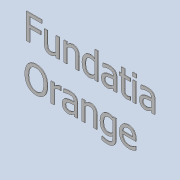
# Autodesk Inventor part: Fundatia orange
Saved by Autodesk Inventor 2020 (Build 240168000, 168)
## iProperties
Created: 2021-01-22
Part Number: Fundatia orange
Material: Generic
Document SubType Name: Modeling
Designer: Iulian Bors
Density: 1 g/cm^3
Appearance: Default
Author: Iulian Bors
Autodesk Inventor part; units mm, degrees
ref_plane "YZ Plane" through (0, 0, 0) normal (1, 0, 0) x (0, 1, 0)
ref_plane "XZ Plane" through (0, 0, 0) normal (0, 1, 0) x (-1, 0, 0)
ref_plane "XY Plane" through (0, 0, 0) normal (0, 0, 1) x (1, 0, 0)
sketch "Sketch1" plane through (0, 0, 0) normal (0, 0, 1) x (1, 0, 0)
  line L0 (-100, 150) -> (100, 150)
  line L1 (100, 150) -> (100, -150)
  line L2 (100, -150) -> (-100, -150)
  line L3 (-100, -150) -> (-100, 150)
  line L4 (-64.214, 58.4793) -> (-50.2905, 58.4793) construction
  line L5 (-50.2905, 58.4793) -> (-50.2905, 44.5299) construction
  line L6 (-50.2905, 44.5299) -> (-64.214, 44.5299) construction
  line L7 (-64.214, 44.5299) -> (-64.214, 58.4793) construction
  line L8 (-25, -80) -> (25, -80)
  line L9 (25, -80) -> (25, -130)
  line L10 (25, -130) -> (-25, -130)
  line L11 (-25, -130) -> (-25, -80)
  line L12 (-46.7302, 54.4072) -> (-58.359, 54.4072)
  line L13 (-58.359, 54.4072) -> (-58.359, 47.357)
  line L14 (-58.359, 47.357) -> (-47.2164, 47.357)
  line L15 (-47.2164, 47.357) -> (-47.2164, 44.3991)
  line L16 (-47.2164, 44.3991) -> (-58.359, 44.3991)
  line L17 (-58.359, 44.3991) -> (-58.359, 32.3651)
  line L18 (-58.359, 32.3651) -> (-61.6815, 32.3651)
  line L19 (-61.6815, 32.3651) -> (-61.6815, 57.3651)
  line L20 (-61.6815, 57.3651) -> (-46.7302, 57.3651)
  line L21 (-46.7302, 57.3651) -> (-46.7302, 54.4072)
  line L22 (-29.4084, 32.3651) -> (-32.5689, 32.3651)
  line L23 (-32.5689, 32.3651) -> (-32.5689, 34.4315)
  spline S0 degree 2 poles (-32.5689, 34.4315) (-34.0276, 33.1552) (-36.641, 31.8383) (-38.2618, 31.8383) knots 0 0 0 1 2 2 2
  spline S1 degree 2 poles (-38.2618, 31.8383) (-39.4773, 31.8383) (-41.6451, 32.6487) (-42.4352, 33.5199) knots 0 0 0 1 2 2 2
  spline S2 degree 2 poles (-42.4352, 33.5199) (-43.2456, 34.391) (-44.137, 37.045) (-44.137, 38.9494) knots 0 0 0 1 2 2 2
  line L24 (-44.137, 38.9494) -> (-44.137, 51.1252)
  line L25 (-44.137, 51.1252) -> (-40.9765, 51.1252)
  line L26 (-40.9765, 51.1252) -> (-40.9765, 40.4283)
  spline S3 degree 2 poles (-40.9765, 40.4283) (-40.9765, 38.9291) (-40.7537, 36.9639) (-40.3687, 36.2346) knots 0 0 0 1 2 2 2
  spline S4 degree 2 poles (-40.3687, 36.2346) (-39.9838, 35.5053) (-38.667, 34.8367) (-37.4311, 34.8367) knots 0 0 0 1 2 2 2
  spline S5 degree 2 poles (-37.4311, 34.8367) (-36.2764, 34.8367) (-33.6629, 36.1536) (-32.5689, 37.1058) knots 0 0 0 1 2 2 2
  line L27 (-32.5689, 37.1058) -> (-32.5689, 51.1252)
  line L28 (-32.5689, 51.1252) -> (-29.4084, 51.1252)
  line L29 (-29.4084, 51.1252) -> (-29.4084, 32.3651)
  line L30 (-10.1013, 32.3651) -> (-13.2618, 32.3651)
  line L31 (-13.2618, 32.3651) -> (-13.2618, 43.062)
  spline S6 degree 2 poles (-13.2618, 43.062) (-13.2618, 44.3586) (-13.5049, 46.5871) (-13.8696, 47.2557) knots 0 0 0 1 2 2 2
  spline S7 degree 2 poles (-13.8696, 47.2557) (-14.2545, 47.9648) (-15.6321, 48.6536) (-16.8072, 48.6536) knots 0 0 0 1 2 2 2
  spline S8 degree 2 poles (-16.8072, 48.6536) (-17.9822, 48.6536) (-20.4741, 47.3975) (-21.6694, 46.3845) knots 0 0 0 1 2 2 2
  line L32 (-21.6694, 46.3845) -> (-21.6694, 32.3651)
  line L33 (-21.6694, 32.3651) -> (-24.8298, 32.3651)
  line L34 (-24.8298, 32.3651) -> (-24.8298, 51.1252)
  line L35 (-24.8298, 51.1252) -> (-21.6694, 51.1252)
  line L36 (-21.6694, 51.1252) -> (-21.6694, 49.0385)
  spline S9 degree 2 poles (-21.6694, 49.0385) (-20.2512, 50.3148) (-17.5162, 51.652) (-15.9765, 51.652) knots 0 0 0 1 2 2 2
  spline S10 degree 2 poles (-15.9765, 51.652) (-13.2213, 51.652) (-10.1013, 48.0053) (-10.1013, 44.5409) knots 0 0 0 1 2 2 2
  line L37 (-10.1013, 44.5409) -> (-10.1013, 32.3651)
  line L38 (8.7601, 32.3651) -> (5.5997, 32.3651)
  line L39 (5.5997, 32.3651) -> (5.5997, 34.2695)
  spline S11 degree 2 poles (5.5997, 34.2695) (4.8703, 33.6617) (3.7966, 32.8513) (3.0672, 32.5069) knots 0 0 0 1 2 2 2
  spline S12 degree 2 poles (3.0672, 32.5069) (2.3987, 32.1827) (0.9603, 31.8383) (0.0081, 31.8383) knots 0 0 0 1 2 2 2
  spline S13 degree 2 poles (0.0081, 31.8383) (-1.5316, 31.8383) (-4.1248, 33.1147) (-5.0365, 34.3505) knots 0 0 0 1 2 2 2
  spline S14 degree 2 poles (-5.0365, 34.3505) (-5.9482, 35.5863) (-6.9611, 39.233) (-6.9611, 41.6033) knots 0 0 0 1 2 2 2
  spline S15 degree 2 poles (-6.9611, 41.6033) (-6.9611, 44.075) (-5.6848, 47.6811) (-4.5705, 49.0385) knots 0 0 0 1 2 2 2
  spline S16 degree 2 poles (-4.5705, 49.0385) (-3.5373, 50.2541) (-0.6402, 51.652) (0.9603, 51.652) knots 0 0 0 1 2 2 2
  spline S17 degree 2 poles (0.9603, 51.652) (2.3582, 51.652) (4.4449, 51.0239) (5.5997, 50.3756) knots 0 0 0 1 2 2 2
  line L40 (5.5997, 50.3756) -> (5.5997, 58.4793)
  line L41 (5.5997, 58.4793) -> (8.7601, 58.4793)
  line L42 (8.7601, 58.4793) -> (8.7601, 32.3651)
  line L43 (5.5997, 36.9234) -> (5.5997, 47.7622)
  spline S18 degree 2 poles (5.5997, 47.7622) (4.4246, 48.3294) (2.5608, 48.7549) (1.487, 48.7549) knots 0 0 0 1 2 2 2
  spline S19 degree 2 poles (1.487, 48.7549) (-0.9441, 48.7549) (-3.6994, 45.1082) (-3.6994, 41.6641) knots 0 0 0 1 2 2 2
  spline S20 degree 2 poles (-3.6994, 41.6641) (-3.6994, 38.3416) (-1.5924, 34.8367) (0.7374, 34.8367) knots 0 0 0 1 2 2 2
  spline S21 degree 2 poles (0.7374, 34.8367) (1.9732, 34.8367) (4.4854, 35.9712) (5.5997, 36.9234) knots 0 0 0 1 2 2 2
  spline S22 degree 2 poles (23.7925, 34.3505) (23.4076, 34.0669) (22.111, 33.0539) (21.5032, 32.75) knots 0 0 0 1 2 2 2
  spline S23 degree 2 poles (21.5032, 32.75) (20.6726, 32.3043) (19.1126, 31.8383) (17.6945, 31.8383) knots 0 0 0 1 2 2 2
  spline S24 degree 2 poles (17.6945, 31.8383) (16.5397, 31.8383) (14.453, 32.7095) (13.6629, 33.4996) knots 0 0 0 1 2 2 2
  spline S25 degree 2 poles (13.6629, 33.4996) (12.9133, 34.2695) (12.0016, 36.5385) (12.0016, 37.7946) knots 0 0 0 1 2 2 2
  spline S26 degree 2 poles (12.0016, 37.7946) (12.0016, 39.7395) (13.6426, 42.4947) (15.4254, 43.2849) knots 0 0 0 1 2 2 2
  spline S27 degree 2 poles (15.4254, 43.2849) (17.0057, 44.0142) (21.3006, 44.5612) (23.7925, 44.703) knots 0 0 0 1 2 2 2
  line L44 (23.7925, 44.703) -> (23.7925, 45.3108)
  spline S28 degree 2 poles (23.7925, 45.3108) (23.7925, 46.4048) (23.124, 47.7622) (22.5162, 48.1471) knots 0 0 0 1 2 2 2
  spline S29 degree 2 poles (22.5162, 48.1471) (21.9084, 48.532) (20.1661, 48.7751) (19.2342, 48.7751) knots 0 0 0 1 2 2 2
  spline S30 degree 2 poles (19.2342, 48.7751) (18.1402, 48.7751) (15.1823, 48.1268) (13.7034, 47.4988) knots 0 0 0 1 2 2 2
  line L45 (13.7034, 47.4988) -> (13.521, 47.4988)
  line L46 (13.521, 47.4988) -> (13.521, 50.72)
  spline S31 degree 2 poles (13.521, 50.72) (14.3922, 50.9631) (17.6539, 51.5709) (19.2544, 51.5709) knots 0 0 0 1 2 2 2
  spline S32 degree 2 poles (19.2544, 51.5709) (21.1993, 51.5709) (23.8533, 50.9631) (24.9068, 50.173) knots 0 0 0 1 2 2 2
  spline S33 degree 2 poles (24.9068, 50.173) (25.94, 49.4032) (26.953, 46.9518) (26.953, 45.1892) knots 0 0 0 1 2 2 2
  line L47 (26.953, 45.1892) -> (26.953, 32.3651)
  line L48 (26.953, 32.3651) -> (23.7925, 32.3651)
  line L49 (23.7925, 32.3651) -> (23.7925, 34.3505)
  line L50 (23.7925, 36.9842) -> (23.7925, 42.1908)
  spline S34 degree 2 poles (23.7925, 42.1908) (22.658, 42.0896) (19.2342, 41.7451) (18.1604, 41.421) knots 0 0 0 1 2 2 2
  spline S35 degree 2 poles (18.1604, 41.421) (16.9044, 41.0361) (15.2634, 39.4356) (15.2634, 38.0174) knots 0 0 0 1 2 2 2
  spline S36 degree 2 poles (15.2634, 38.0174) (15.2634, 36.3967) (17.0867, 34.7557) (18.829, 34.7557) knots 0 0 0 1 2 2 2
  spline S37 degree 2 poles (18.829, 34.7557) (20.3079, 34.7557) (22.739, 36.032) (23.7925, 36.9842) knots 0 0 0 1 2 2 2
  spline S38 degree 2 poles (37.0624, 32.0004) (34.4894, 32.0004) (31.5924, 34.938) (31.5924, 38.1187) knots 0 0 0 1 2 2 2
  line L51 (31.5924, 38.1187) -> (31.5924, 48.5118)
  line L52 (31.5924, 48.5118) -> (29.4651, 48.5118)
  line L53 (29.4651, 48.5118) -> (29.4651, 51.1252)
  line L54 (29.4651, 51.1252) -> (31.5924, 51.1252)
  line L55 (31.5924, 51.1252) -> (31.5924, 56.5142)
  line L56 (31.5924, 56.5142) -> (34.7528, 56.5142)
  line L57 (34.7528, 56.5142) -> (34.7528, 51.1252)
  line L58 (34.7528, 51.1252) -> (40.5672, 51.1252)
  line L59 (40.5672, 51.1252) -> (40.5672, 48.5118)
  line L60 (40.5672, 48.5118) -> (34.7528, 48.5118)
  line L61 (34.7528, 48.5118) -> (34.7528, 39.5774)
  spline S39 degree 2 poles (34.7528, 39.5774) (34.7528, 38.1592) (34.8541, 36.5993) (35.1985, 35.9307) knots 0 0 0 1 2 2 2
  spline S40 degree 2 poles (35.1985, 35.9307) (35.4822, 35.3432) (36.7585, 34.7557) (37.8525, 34.7557) knots 0 0 0 1 2 2 2
  spline S41 degree 2 poles (37.8525, 34.7557) (38.6223, 34.7557) (40.0608, 35.2216) (40.3849, 35.3635) knots 0 0 0 1 2 2 2
  line L62 (40.3849, 35.3635) -> (40.5672, 35.3635)
  line L63 (40.5672, 35.3635) -> (40.5672, 32.5272)
  spline S42 degree 2 poles (40.5672, 32.5272) (39.6758, 32.284) (37.8525, 32.0004) (37.0624, 32.0004) knots 0 0 0 1 2 2 2
  line L64 (46.1183, 32.3651) -> (42.9578, 32.3651)
  line L65 (42.9578, 32.3651) -> (42.9578, 51.1252)
  line L66 (42.9578, 51.1252) -> (46.1183, 51.1252)
  line L67 (46.1183, 51.1252) -> (46.1183, 32.3651)
  line L68 (46.3411, 54.2451) -> (42.7552, 54.2451)
  line L69 (42.7552, 54.2451) -> (42.7552, 57.5272)
  line L70 (42.7552, 57.5272) -> (46.3411, 57.5272)
  line L71 (46.3411, 57.5272) -> (46.3411, 54.2451)
  spline S43 degree 2 poles (61.2115, 34.3505) (60.8266, 34.0669) (59.53, 33.0539) (58.9222, 32.75) knots 0 0 0 1 2 2 2
  spline S44 degree 2 poles (58.9222, 32.75) (58.0916, 32.3043) (56.5316, 31.8383) (55.1134, 31.8383) knots 0 0 0 1 2 2 2
  spline S45 degree 2 poles (55.1134, 31.8383) (53.9586, 31.8383) (51.8719, 32.7095) (51.0818, 33.4996) knots 0 0 0 1 2 2 2
  spline S46 degree 2 poles (51.0818, 33.4996) (50.3322, 34.2695) (49.4206, 36.5385) (49.4206, 37.7946) knots 0 0 0 1 2 2 2
  spline S47 degree 2 poles (49.4206, 37.7946) (49.4206, 39.7395) (51.0616, 42.4947) (52.8444, 43.2849) knots 0 0 0 1 2 2 2
  spline S48 degree 2 poles (52.8444, 43.2849) (54.4246, 44.0142) (58.7196, 44.5612) (61.2115, 44.703) knots 0 0 0 1 2 2 2
  line L72 (61.2115, 44.703) -> (61.2115, 45.3108)
  spline S49 degree 2 poles (61.2115, 45.3108) (61.2115, 46.4048) (60.5429, 47.7622) (59.9351, 48.1471) knots 0 0 0 1 2 2 2
  spline S50 degree 2 poles (59.9351, 48.1471) (59.3274, 48.532) (57.5851, 48.7751) (56.6531, 48.7751) knots 0 0 0 1 2 2 2
  spline S51 degree 2 poles (56.6531, 48.7751) (55.5591, 48.7751) (52.6013, 48.1268) (51.1223, 47.4988) knots 0 0 0 1 2 2 2
  line L73 (51.1223, 47.4988) -> (50.94, 47.4988)
  line L74 (50.94, 47.4988) -> (50.94, 50.72)
  spline S52 degree 2 poles (50.94, 50.72) (51.8112, 50.9631) (55.0729, 51.5709) (56.6734, 51.5709) knots 0 0 0 1 2 2 2
  spline S53 degree 2 poles (56.6734, 51.5709) (58.6183, 51.5709) (61.2723, 50.9631) (62.3257, 50.173) knots 0 0 0 1 2 2 2
  spline S54 degree 2 poles (62.3257, 50.173) (63.359, 49.4032) (64.3719, 46.9518) (64.3719, 45.1892) knots 0 0 0 1 2 2 2
  line L75 (64.3719, 45.1892) -> (64.3719, 32.3651)
  line L76 (64.3719, 32.3651) -> (61.2115, 32.3651)
  line L77 (61.2115, 32.3651) -> (61.2115, 34.3505)
  line L78 (61.2115, 36.9842) -> (61.2115, 42.1908)
  spline S55 degree 2 poles (61.2115, 42.1908) (60.077, 42.0896) (56.6531, 41.7451) (55.5794, 41.421) knots 0 0 0 1 2 2 2
  spline S56 degree 2 poles (55.5794, 41.421) (54.3233, 41.0361) (52.6823, 39.4356) (52.6823, 38.0174) knots 0 0 0 1 2 2 2
  spline S57 degree 2 poles (52.6823, 38.0174) (52.6823, 36.3967) (54.5057, 34.7557) (56.248, 34.7557) knots 0 0 0 1 2 2 2
  spline S58 degree 2 poles (56.248, 34.7557) (57.7269, 34.7557) (60.158, 36.032) (61.2115, 36.9842) knots 0 0 0 1 2 2 2
  spline S59 degree 2 poles (-43.9952, 13.3467) (-42.577, 11.6854) (-40.9968, 6.8232) (-40.9968, 3.7032) knots 0 0 0 1 2 2 2
  spline S60 degree 2 poles (-40.9968, 3.7032) (-40.9968, 0.6643) (-42.5365, -4.2587) (-43.9952, -5.9199) knots 0 0 0 1 2 2 2
  spline S61 degree 2 poles (-43.9952, -5.9199) (-45.5349, -7.6622) (-49.607, -9.3235) (-52.0584, -9.3235) knots 0 0 0 1 2 2 2
  spline S62 degree 2 poles (-52.0584, -9.3235) (-54.5908, -9.3235) (-58.6426, -7.6015) (-60.1216, -5.9199) knots 0 0 0 1 2 2 2
  spline S63 degree 2 poles (-60.1216, -5.9199) (-61.56, -4.2587) (-63.0997, 0.6238) (-63.0997, 3.7032) knots 0 0 0 1 2 2 2
  spline S64 degree 2 poles (-63.0997, 3.7032) (-63.0997, 6.8434) (-61.5397, 11.6246) (-60.1013, 13.3467) knots 0 0 0 1 2 2 2
  spline S65 degree 2 poles (-60.1013, 13.3467) (-58.6426, 15.0079) (-54.5705, 16.73) (-52.0584, 16.73) knots 0 0 0 1 2 2 2
  spline S66 degree 2 poles (-52.0584, 16.73) (-49.5057, 16.73) (-45.4133, 14.9472) (-43.9952, 13.3467) knots 0 0 0 1 2 2 2
  spline S67 degree 2 poles (-44.4611, 3.7032) (-44.4611, 6.1749) (-45.5349, 10.0039) (-46.5073, 11.26) knots 0 0 0 1 2 2 2
  spline S68 degree 2 poles (-46.5073, 11.26) (-47.5, 12.5566) (-50.2958, 13.8532) (-52.0381, 13.8532) knots 0 0 0 1 2 2 2
  spline S69 degree 2 poles (-52.0381, 13.8532) (-53.8412, 13.8532) (-56.5559, 12.5971) (-57.5892, 11.26) knots 0 0 0 1 2 2 2
  spline S70 degree 2 poles (-57.5892, 11.26) (-58.5819, 9.9836) (-59.6354, 6.1344) (-59.6354, 3.7032) knots 0 0 0 1 2 2 2
  spline S71 degree 2 poles (-59.6354, 3.7032) (-59.6354, -1.2198) (-55.5025, -6.4467) (-52.0381, -6.4467) knots 0 0 0 1 2 2 2
  spline S72 degree 2 poles (-52.0381, -6.4467) (-48.5738, -6.4467) (-44.4611, -1.2198) (-44.4611, 3.7032) knots 0 0 0 1 2 2 2
  line L79 (-27.6459, 6.5801) -> (-27.808, 6.5801)
  spline S73 degree 2 poles (-27.808, 6.5801) (-28.1726, 6.6814) (-28.9627, 6.7219) (-29.5097, 6.7219) knots 0 0 0 1 2 2 2
  spline S74 degree 2 poles (-29.5097, 6.7219) (-30.7861, 6.7219) (-33.2982, 5.6076) (-34.4328, 4.5136) knots 0 0 0 1 2 2 2
  line L80 (-34.4328, 4.5136) -> (-34.4328, -8.7968)
  line L81 (-34.4328, -8.7968) -> (-37.5932, -8.7968)
  line L82 (-37.5932, -8.7968) -> (-37.5932, 9.9634)
  line L83 (-37.5932, 9.9634) -> (-34.4328, 9.9634)
  line L84 (-34.4328, 9.9634) -> (-34.4328, 7.1676)
  spline S75 degree 2 poles (-34.4328, 7.1676) (-32.7107, 8.7073) (-30.1378, 9.9634) (-28.9222, 9.9634) knots 0 0 0 1 2 2 2
  spline S76 degree 2 poles (-28.9222, 9.9634) (-28.436, 9.9634) (-27.9498, 9.9228) (-27.6459, 9.8621) knots 0 0 0 1 2 2 2
  line L85 (-27.6459, 9.8621) -> (-27.6459, 6.5801)
  spline S77 degree 2 poles (-14.7407, -6.8113) (-15.1256, -7.095) (-16.4222, -8.1079) (-17.03, -8.4118) knots 0 0 0 1 2 2 2
  spline S78 degree 2 poles (-17.03, -8.4118) (-17.8606, -8.8575) (-19.4206, -9.3235) (-20.8388, -9.3235) knots 0 0 0 1 2 2 2
  spline S79 degree 2 poles (-20.8388, -9.3235) (-21.9935, -9.3235) (-24.0802, -8.4524) (-24.8704, -7.6622) knots 0 0 0 1 2 2 2
  spline S80 degree 2 poles (-24.8704, -7.6622) (-25.62, -6.8924) (-26.5316, -4.6233) (-26.5316, -3.3673) knots 0 0 0 1 2 2 2
  spline S81 degree 2 poles (-26.5316, -3.3673) (-26.5316, -1.4224) (-24.8906, 1.3329) (-23.1078, 2.123) knots 0 0 0 1 2 2 2
  spline S82 degree 2 poles (-23.1078, 2.123) (-21.5276, 2.8523) (-17.2326, 3.3993) (-14.7407, 3.5412) knots 0 0 0 1 2 2 2
  line L86 (-14.7407, 3.5412) -> (-14.7407, 4.1489)
  spline S83 degree 2 poles (-14.7407, 4.1489) (-14.7407, 5.2429) (-15.4093, 6.6003) (-16.017, 6.9852) knots 0 0 0 1 2 2 2
  spline S84 degree 2 poles (-16.017, 6.9852) (-16.6248, 7.3702) (-18.3671, 7.6133) (-19.299, 7.6133) knots 0 0 0 1 2 2 2
  spline S85 degree 2 poles (-19.299, 7.6133) (-20.3931, 7.6133) (-23.3509, 6.965) (-24.8298, 6.3369) knots 0 0 0 1 2 2 2
  line L87 (-24.8298, 6.3369) -> (-25.0122, 6.3369)
  line L88 (-25.0122, 6.3369) -> (-25.0122, 9.5582)
  spline S86 degree 2 poles (-25.0122, 9.5582) (-24.141, 9.8013) (-20.8793, 10.4091) (-19.2788, 10.4091) knots 0 0 0 1 2 2 2
  spline S87 degree 2 poles (-19.2788, 10.4091) (-17.3339, 10.4091) (-14.6799, 9.8013) (-13.6264, 9.0112) knots 0 0 0 1 2 2 2
  spline S88 degree 2 poles (-13.6264, 9.0112) (-12.5932, 8.2413) (-11.5802, 5.7899) (-11.5802, 4.0274) knots 0 0 0 1 2 2 2
  line L89 (-11.5802, 4.0274) -> (-11.5802, -8.7968)
  line L90 (-11.5802, -8.7968) -> (-14.7407, -8.7968)
  line L91 (-14.7407, -8.7968) -> (-14.7407, -6.8113)
  line L92 (-14.7407, -4.1776) -> (-14.7407, 1.029)
  spline S89 degree 2 poles (-14.7407, 1.029) (-15.8752, 0.9277) (-19.299, 0.5833) (-20.3728, 0.2592) knots 0 0 0 1 2 2 2
  spline S90 degree 2 poles (-20.3728, 0.2592) (-21.6289, -0.1258) (-23.2699, -1.7263) (-23.2699, -3.1444) knots 0 0 0 1 2 2 2
  spline S91 degree 2 poles (-23.2699, -3.1444) (-23.2699, -4.7652) (-21.4465, -6.4062) (-19.7042, -6.4062) knots 0 0 0 1 2 2 2
  spline S92 degree 2 poles (-19.7042, -6.4062) (-18.2253, -6.4062) (-15.7942, -5.1298) (-14.7407, -4.1776) knots 0 0 0 1 2 2 2
  line L93 (7.5851, -8.7968) -> (4.4246, -8.7968)
  line L94 (4.4246, -8.7968) -> (4.4246, 1.9002)
  spline S93 degree 2 poles (4.4246, 1.9002) (4.4246, 3.1968) (4.1815, 5.4253) (3.8168, 6.0938) knots 0 0 0 1 2 2 2
  spline S94 degree 2 poles (3.8168, 6.0938) (3.4319, 6.8029) (2.0543, 7.4917) (0.8792, 7.4917) knots 0 0 0 1 2 2 2
  spline S95 degree 2 poles (0.8792, 7.4917) (-0.2958, 7.4917) (-2.7877, 6.2357) (-3.983, 5.2227) knots 0 0 0 1 2 2 2
  line L95 (-3.983, 5.2227) -> (-3.983, -8.7968)
  line L96 (-3.983, -8.7968) -> (-7.1435, -8.7968)
  line L97 (-7.1435, -8.7968) -> (-7.1435, 9.9634)
  line L98 (-7.1435, 9.9634) -> (-3.983, 9.9634)
  line L99 (-3.983, 9.9634) -> (-3.983, 7.8767)
  spline S96 degree 2 poles (-3.983, 7.8767) (-2.5649, 9.153) (0.1702, 10.4901) (1.7099, 10.4901) knots 0 0 0 1 2 2 2
  spline S97 degree 2 poles (1.7099, 10.4901) (4.4651, 10.4901) (7.5851, 6.8434) (7.5851, 3.3791) knots 0 0 0 1 2 2 2
  line L100 (7.5851, 3.3791) -> (7.5851, -8.7968)
  spline S98 degree 2 poles (12.6904, -11.7951) (13.0146, -11.937) (14.2504, -12.3827) (15.0405, -12.565) knots 0 0 0 1 2 2 2
  spline S99 degree 2 poles (15.0405, -12.565) (15.9116, -12.7878) (17.3906, -13.0512) (18.2617, -13.0512) knots 0 0 0 1 2 2 2
  spline S100 degree 2 poles (18.2617, -13.0512) (19.7204, -13.0512) (21.7463, -12.2814) (22.3136, -11.5925) knots 0 0 0 1 2 2 2
  spline S101 degree 2 poles (22.3136, -11.5925) (22.8606, -10.9037) (23.286, -9.1007) (23.286, -7.9459) knots 0 0 0 1 2 2 2
  line L101 (23.286, -7.9459) -> (23.286, -6.3049)
  spline S102 degree 2 poles (23.286, -6.3049) (22.0097, -7.4191) (19.5583, -8.4726) (17.7147, -8.4726) knots 0 0 0 1 2 2 2
  spline S103 degree 2 poles (17.7147, -8.4726) (14.5138, -8.4726) (10.7253, -3.7117) (10.7253, 0.7656) knots 0 0 0 1 2 2 2
  spline S104 degree 2 poles (10.7253, 0.7656) (10.7253, 3.0955) (12.0421, 6.7016) (13.1361, 7.978) knots 0 0 0 1 2 2 2
  spline S105 degree 2 poles (13.1361, 7.978) (14.1896, 9.1733) (17.0867, 10.4901) (18.6264, 10.4901) knots 0 0 0 1 2 2 2
  spline S106 degree 2 poles (18.6264, 10.4901) (20.0851, 10.4901) (22.2123, 9.8013) (23.286, 9.1733) knots 0 0 0 1 2 2 2
  line L102 (23.286, 9.1733) -> (23.4684, 9.9634)
  line L103 (23.4684, 9.9634) -> (26.4465, 9.9634)
  line L104 (26.4465, 9.9634) -> (26.4465, -6.6493)
  spline S107 degree 2 poles (26.4465, -6.6493) (26.4465, -11.4305) (22.2933, -15.8875) (18.0186, -15.8875) knots 0 0 0 1 2 2 2
  spline S108 degree 2 poles (18.0186, -15.8875) (16.641, -15.8875) (13.7642, -15.4418) (12.5283, -15.0772) knots 0 0 0 1 2 2 2
  line L105 (12.5283, -15.0772) -> (12.5283, -11.7951)
  line L106 (12.5283, -11.7951) -> (12.6904, -11.7951)
  line L107 (23.286, -3.7117) -> (23.286, 6.6003)
  spline S109 degree 2 poles (23.286, 6.6003) (22.111, 7.1676) (20.1256, 7.6538) (19.1329, 7.6538) knots 0 0 0 1 2 2 2
  spline S110 degree 2 poles (19.1329, 7.6538) (16.7423, 7.6538) (13.987, 4.1287) (13.987, 0.8264) knots 0 0 0 1 2 2 2
  spline S111 degree 2 poles (13.987, 0.8264) (13.987, -2.2935) (16.0737, -5.5553) (18.4238, -5.5553) knots 0 0 0 1 2 2 2
  spline S112 degree 2 poles (18.4238, -5.5553) (19.6596, -5.5553) (22.2528, -4.5828) (23.286, -3.7117) knots 0 0 0 1 2 2 2
  spline S113 degree 2 poles (39.1693, -9.2222) (34.6718, -9.2222) (29.7285, -4.1776) (29.7285, 0.482) knots 0 0 0 1 2 2 2
  spline S114 degree 2 poles (29.7285, 0.482) (29.7285, 5.0606) (34.53, 10.4901) (38.3995, 10.4901) knots 0 0 0 1 2 2 2
  spline S115 degree 2 poles (38.3995, 10.4901) (40.1418, 10.4901) (42.8363, 9.4771) (43.829, 8.4034) knots 0 0 0 1 2 2 2
  spline S116 degree 2 poles (43.829, 8.4034) (44.842, 7.3297) (45.9157, 4.23) (45.9157, 1.9812) knots 0 0 0 1 2 2 2
  line L108 (45.9157, 1.9812) -> (45.9157, 0.2592)
  line L109 (45.9157, 0.2592) -> (32.9295, 0.2592)
  spline S117 degree 2 poles (32.9295, 0.2592) (32.9295, -3.0026) (36.2115, -6.4669) (39.1288, -6.4669) knots 0 0 0 1 2 2 2
  spline S118 degree 2 poles (39.1288, -6.4669) (40.1621, -6.4669) (42.1677, -6.001) (42.9781, -5.6363) knots 0 0 0 1 2 2 2
  spline S119 degree 2 poles (42.9781, -5.6363) (43.829, -5.2311) (45.004, -4.522) (45.389, -4.1979) knots 0 0 0 1 2 2 2
  line L110 (45.389, -4.1979) -> (45.5713, -4.1979)
  line L111 (45.5713, -4.1979) -> (45.5713, -7.642)
  spline S120 degree 2 poles (45.5713, -7.642) (45.0243, -7.8648) (43.363, -8.5131) (42.7147, -8.6955) knots 0 0 0 1 2 2 2
  spline S121 degree 2 poles (42.7147, -8.6955) (41.8031, -8.9588) (40.3039, -9.2222) (39.1693, -9.2222) knots 0 0 0 1 2 2 2
  spline S122 degree 2 poles (42.8363, 2.67) (42.7958, 3.9463) (42.269, 5.8102) (41.7625, 6.4382) knots 0 0 0 1 2 2 2
  spline S123 degree 2 poles (41.7625, 6.4382) (41.2155, 7.1473) (39.4935, 7.8969) (38.2172, 7.8969) knots 0 0 0 1 2 2 2
  spline S124 degree 2 poles (38.2172, 7.8969) (36.9611, 7.8969) (35.1985, 7.1473) (34.4692, 6.418) knots 0 0 0 1 2 2 2
  spline S125 degree 2 poles (34.4692, 6.418) (33.7601, 5.6684) (33.0308, 3.8653) (32.9295, 2.67) knots 0 0 0 1 2 2 2
  line L112 (32.9295, 2.67) -> (42.8363, 2.67)
  point P0 (0, 0)
  point P1 (0, 150)
  point P2 (-100, 0)
  point P3 (0, -130)
  point P4 (0, -150)
  dimension "d0" = 300
  dimension "d1" = 200
  dimension "d4" = 50
  dimension "d5" = 50
  dimension "d6" = 20
  constraints: 16 end point, 4 midpoint, 4 parallel, 2 horizontal, 2 perpendicular, 2 vertical alignment, 1 horizontal alignment, 2 other
  measures "d0" distance of L2.end L0.start
  measures "d1" distance of L1.end L2.end
  measures "d4" distance of L8.start L8.end
  measures "d5" distance of L8.end L9.end
  measures "d6" distance between parallel lines of L2 L10
extrude "Extrusion1" add sketch "Sketch1" along normal blind 0.6 contours L12 L13 L14 L15 L16 L17 L18 L19 L20 L21 | L22 L23 S0 S1 S2 L24 L25 L26 S3 S4 S5 L27 L28 L29 | L30 L31 S6 S7 S8 L32 L33 L34 L35 L36 S9 S10 L37 | L38 L39 S11 S12 S13 S14 S15 S16 S17 L40 L41 L42 | S22 S23 S24 S25 S26 S27 L44 S28 S29 S30 L45 L46 S31 S32 S33 L47 L48 L49 | S38 L51 L52 L53 L54 L55 L56 L57 L58 L59 L60 L61 S39 S40 S41 L62 L63 S42 | L64 L65 L66 L67 | L68 L69 L70 L71 | S43 S44 S45 S46 S47 S48 L72 S49 S50 S51 L73 L74 S52 S53 S54 L75 L76 L77 | S59 S60 S61 S62 S63 S64 S65 S66 | L79 S73 S74 L80 L81 L82 L83 L84 S75 S76 L85 | S77 S78 S79 S80 S81 S82 L86 S83 S84 S85 L87 L88 S86 S87 S88 L89 L90 L91 | L93 L94 S93 S94 S95 L95 L96 L97 L98 L99 S96 S97 L100 | S98 S99 S100 S101 L101 S102 S103 S104 S105 S106 L102 L103 L104 S107 S108 L105 L106 | S113 S114 S115 S116 L108 L109 S117 S118 S119 L110 L111 S120 S121
body "Solid1"
